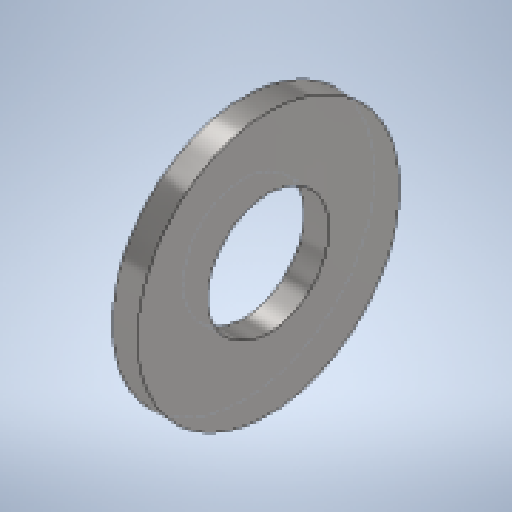
# Autodesk Inventor part: Needle Bearings
Saved by Autodesk Inventor 2023.2 (Build 272271000, 271)
## iProperties
Created: 2023-08-25
Part Number: Needle Bearings
Material: Steel, Alloy
Document SubType Name: Modeling
Designer: Nathan Cai
Density: 7.73 g/cm^3
Appearance: Semi-Polished
Author: Nathan Cai
Autodesk Inventor part; units mm, degrees
ref_plane "YZ Plane" through (0, 0, 0) normal (1, 0, 0) x (0, 1, 0)
ref_plane "XZ Plane" through (0, 0, 0) normal (0, 1, 0) x (-1, 0, 0)
ref_plane "XY Plane" through (0, 0, 0) normal (0, 0, 1) x (1, 0, 0)
sketch "Sketch1" plane through (0, 0, 0) normal (1, 0, 0) x (0, 1, 0)
  circle A0 centre (0, 0) radius 4.7625
  circle A1 centre (0, 0) radius 10.3188
  dimension "d0" = 9.525
  dimension "d1" = 20.6375
  constraints: 2 centre point, 2 coincident
  measures "d0" diameter of A0
  measures "d1" diameter of A1
extrude "Extrusion1" add sketch "Sketch1" along normal blind 1.9844
body "Solid1"
